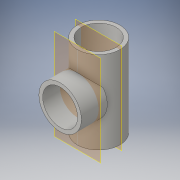
# Autodesk Inventor part: New Elbow
Saved by Autodesk Inventor 2016 (Build 200138000, 138)
## iProperties
Created: 2017-09-22
Part Number: New Elbow
Material: Generic
Document SubType Name: Modeling
Designer: Student
Density: 1 g/cm^3
Appearance: Default
Author: Student
Autodesk Inventor part; units mm, degrees
ref_plane "YZ Plane" through (0, 0, 0) normal (1, 0, 0) x (0, 1, 0)
ref_plane "XZ Plane" through (0, 0, 0) normal (0, 1, 0) x (-1, 0, 0)
sketch "Sketch1" plane through (0, 0, 0) normal (0, 1, 0) x (-1, 0, 0)
  circle A0 centre (0, 0) radius 20.32
  circle A1 centre (0, 0) radius 16.7005
  dimension "d0" = 40.64
  dimension "d1" = 33.401
  constraints: 2 centre point, 2 coincident
  measures "d0" diameter of A0
  measures "d1" diameter of A1
extrude "Extrusion1" add sketch "Sketch1" along normal blind 79.0448
ref_plane "Work Plane1" through (0, 0, 20.32) normal (0, 0, 1) x (1, 0, 0)
sketch "Sketch2" plane through (0, 0, 20.32) normal (0, 0, 1) x (1, 0, 0)
  line L0 (0, 0) -> (0, 79.0448)
  line L1 (20.32, 79.0448) -> (-20.32, 79.0448) projected
  line L2 (-20.32, 0) -> (-20.32, 79.0448) projected
  line L3 (-20.32, 39.5224) -> (20.32, 39.5224)
  line L4 (20.32, 0) -> (20.32, 79.0448) projected
  circle A0 centre (0, 39.5224) radius 16.7005
  circle A1 centre (0, 39.5224) radius 20.32
  dimension "d4" = 33.401
  dimension "d5" = 40.64
  constraints: 4 end point, 4 midpoint, 2 centre point, 1 coincident
  measures "d4" diameter of A0
  measures "d5" diameter of A1
extrude "Extrusion2" add sketch "Sketch2" along normal blind 16.51 and the other way blind 8.255 contours A1 L3 A0 L0 | L0 A0 L3 A1 | A1 L0 A0 L3 | L3 A0 L0 A1
sketch "Sketch3" plane through (0, 39.5224, 36.83) normal (0, 0, 1) x (1, 0, 0)
  circle A0 centre (0, 0) radius 16.7005
  point P0 (0, -39.5224)
  dimension "d10" = 33.401
  constraints: 1 centre point
  measures "d10" diameter of A0
extrude "Extrusion3" cut sketch "Sketch3" against normal blind 25.4
body "Solid1"
